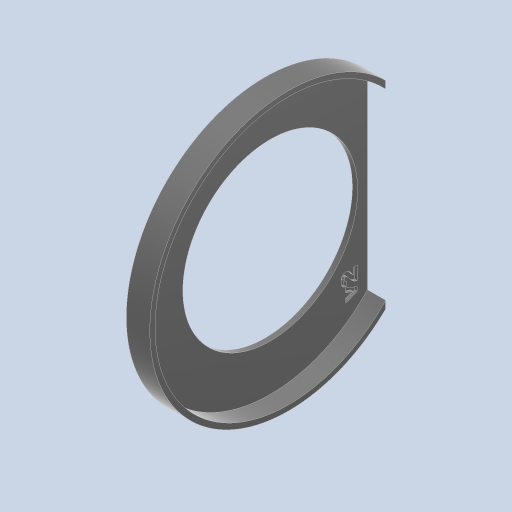
# Autodesk Inventor part: RFID_cover_02
Saved by Autodesk Inventor 2024.4 (Build 284460030, 460C)
## iProperties
Created: 2026-04-27
Part Number: RFID_cover_02
Material: PLA Black
Document SubType Name: Modeling
Designer: tooles01
Density: 1.06 g/cm^3
Appearance: Smooth - White(2)
Author: tooles01
Autodesk Inventor part; units mm, degrees
ref_plane "YZ Plane" through (0, 0, 0) normal (1, 0, 0) x (0, 1, 0)
ref_plane "XZ Plane" through (0, 0, 0) normal (0, 1, 0) x (-1, 0, 0)
ref_plane "XY Plane" through (0, 0, 0) normal (0, 0, 1) x (1, 0, 0)
derived "RFID_holder_coil_01.ipt"
sketch "Sketch2: RFID holder" plane through (0, 0, 0) normal (1, 0, 0) x (0, 0, -1)
  circle A0 centre (-28.125, 0) radius 16.25
  circle A1 centre (-28.125, 0) radius 22
  circle A2 centre (-28.125, 0) radius 24.625
  circle A3 centre (-28.125, 0) radius 25.375
  line L0 (-28.125, 1.5) -> (0, 1.5)
  line L1 (-28.125, -1.5) -> (0, -1.5)
  line L2 (0, -13.4) -> (0, 13.4)
  line L3 (0, -13.4) -> (-3.5, -13.4)
  line L4 (0, 13.4) -> (-3.5, 13.4)
  line L5 (-3.5, 13.4) -> (-3.5, -13.4)
  line L6 (-28.125, 1.5) -> (-28.125, -1.5) construction
  line L7 (-2.75, 13.4) -> (-2.75, -13.4) construction
  line L8 (-1, 13.4) -> (-1, -13.4)
  line L9 (-3.5, -6.1237) -> (0, -6.1237)
  point P0 (0, 0)
  point P1 (-3.5, 0)
  point P2 (0, 0)
sketch "Sketch8: M3 through hole" plane through (0, 0, 0) normal (1, 0, 0) x (0, 1, 0)
  line L0 (20.4, 7) -> (13.4, 7)
  line L1 (13.4, 7) -> (13.4, 0)
  line L2 (13.4, 0) -> (20.4, 0)
  line L3 (20.4, 0) -> (20.4, 7)
  circle A0 centre (16.9, 3.5) radius 1.85
  circle A1 centre (0, 28.125) radius 25.375
  line L4 (13.4, 3.5) -> (-13.4, 3.5)
  line L5 (13.4, 0) -> (13.4, 3.5) construction
  point P0 (0, 0)
  point P1 (20.4, 3.5)
  point P2 (16.9, 7)
sketch "Sketch1: base" plane through (0, 0, 0) normal (1, 0, 0) x (0, 1, 0)
  circle A0 centre (0, 28.125) radius 16.75
  circle A1 centre (0, 28.125) radius 25.575
  circle A2 centre (0, 28.125) radius 26.575
  circle A3 centre (0, 28.125) radius 16.25 construction
  circle A4 centre (0, 28.125) radius 25.375 construction
  line L0 (18.9563, 9.5) -> (-18.9563, 9.5)
  line L1 (13.4, 3.5) -> (-13.4, 3.5) construction
  circle A5 centre (0, 28.125) radius 22 construction
  point P0 (0, 0)
  point P1 (17.5268, 9.5)
  point P2 (-17.5268, 9.5)
  dimension "d2" = 1
  dimension "d4" = 0.2
  dimension "d6" = 6
  dimension "d14" = 0.5
  constraints: 3 centre point, 3 coincident, 2 end point, 2 point on circle, 1 horizontal
  measures "d2" radial gap between concentric circles of A2 A1
  measures "d4" radial gap between concentric circles of A1 A4
  measures "d6" distance between parallel lines of L0 L1
  measures "d14" radial gap between concentric circles of A0 A3
extrude "Ex1: base" add sketch "Sketch1: base" against normal blind 1 contours A1 L0 | A1 L0 A2 picked at (0.673, 10.1657) picked at (-19.3455, 11.1192)
extrude "Ex2: wall" add sketch "Sketch1: base" along normal blind 3.5 contours A1 L0 A2 picked at (-19.3455, 11.1192)
sketch "Sketch:text" plane through (0, 0, 0) normal (1, 0, 0) x (0, 1, 0)
  line L0 (-16.5, 14.5) -> (-13.5, 14.5) construction
  line L1 (-13.5, 14.5) -> (-13.5, 11.5) construction
  line L2 (-13.5, 11.5) -> (-16.5, 11.5) construction
  line L3 (-16.5, 11.5) -> (-16.5, 14.5) construction
  line L4 (-17.7183, 13.659) -> (-16.8376, 13.659)
  line L5 (-16.8376, 13.659) -> (-16.4061, 12.2588)
  line L6 (-16.4061, 12.2588) -> (-15.9628, 13.659)
  line L7 (-15.9628, 13.659) -> (-15.1086, 13.659)
  line L8 (-15.1086, 13.659) -> (-16.048, 11.4486)
  line L9 (-16.048, 11.4486) -> (-16.7995, 11.4486)
  line L10 (-16.7995, 11.4486) -> (-17.7183, 13.659)
  line L11 (-12.4667, 11.4486) -> (-15.0088, 11.4486)
  spline S0 degree 2 poles (-15.0088, 11.4486) (-14.9648, 11.8243) (-14.5215, 12.4878) (-13.9109, 12.9398) knots 0 0 0 1 2 2 2
  spline S1 degree 2 poles (-13.9109, 12.9398) (-13.541, 13.2158) (-13.3326, 13.5034) (-13.3326, 13.6326) knots 0 0 0 1 2 2 2
  spline S2 degree 2 poles (-13.3326, 13.6326) (-13.3326, 13.7735) (-13.5381, 13.9702) (-13.6937, 13.9702) knots 0 0 0 1 2 2 2
  spline S3 degree 2 poles (-13.6937, 13.9702) (-13.8581, 13.9702) (-14.0636, 13.7676) (-14.0988, 13.5093) knots 0 0 0 1 2 2 2
  line L12 (-14.0988, 13.5093) -> (-14.9472, 13.5768)
  spline S4 degree 2 poles (-14.9472, 13.5768) (-14.8973, 13.935) (-14.6301, 14.3371) (-14.1458, 14.5514) (-13.7172, 14.5514) knots 0 0 0 1 2 3 3 3
  spline S5 degree 2 poles (-13.7172, 14.5514) (-13.271, 14.5514) (-12.7719, 14.3459) (-12.4872, 13.9262) (-12.4872, 13.662) knots 0 0 0 1 2 3 3 3
  spline S6 degree 2 poles (-12.4872, 13.662) (-12.4872, 13.3831) (-12.813, 12.8752) (-13.2446, 12.5699) knots 0 0 0 1 2 2 2
  spline S7 degree 2 poles (-13.2446, 12.5699) (-13.5, 12.3938) (-13.6731, 12.2529) (-13.7906, 12.1384) knots 0 0 0 1 2 2 2
  line L13 (-13.7906, 12.1384) -> (-12.4667, 12.1384)
  line L14 (-12.4667, 12.1384) -> (-12.4667, 11.4486)
  point P0 (0, 0)
  point P1 (-15, 11.5)
  point P2 (-13.5, 13)
  dimension "d15" = 3
  dimension "d16" = 13
  dimension "d17" = 15
  constraints: 2 midpoint, 1 horizontal, 1 perpendicular, 2 other
  measures "d15" distance of L0.start L0.end
  measures "d16" vertical distance of point (0, 0) point (-13.5, 13)
  measures "d17" horizontal distance of point (0, 0) point (-15, 11.5)
extrude "Ex: text" cut sketch "Sketch:text" against normal blind 0.5
fillet "Fillet1" [suppressed]
fillet "Fillet2" [suppressed]
fillet "Fillet3" [suppressed]
body "Solid2"
